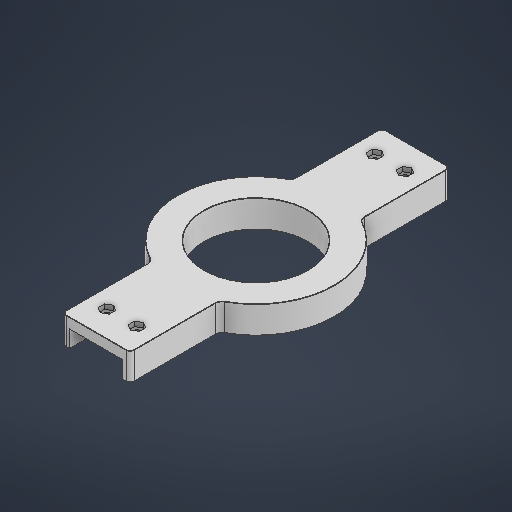
# Autodesk Inventor part: Head Thing
Saved by Autodesk Inventor 2025 (Build 290162000, 162)
## iProperties
Created: 2024-04-28
Part Number: Head Thing
Material: Generic
Document SubType Name: Modeling
Designer: Thienan Hoang
Density: 1 g/cm^3
Appearance: Default
Author: Thienan Hoang
Autodesk Inventor part; units mm, degrees
ref_plane "YZ Plane" through (0, 0, 0) normal (1, 0, 0) x (0, 1, 0)
ref_plane "XZ Plane" through (0, 0, 0) normal (0, 1, 0) x (-1, 0, 0)
ref_plane "XY Plane" through (0, 0, 0) normal (0, 0, 1) x (1, 0, 0)
sketch "Sketch1" plane through (0, 0, 0) normal (0, 1, 0) x (-1, 0, 0)
  circle A0 centre (0, 0) radius 38.125
  line L0 (25, 117.5) -> (-25, 117.5)
  line L1 (-25, -117.5) -> (25, -117.5)
  arc A1 (-25, 51.7808) -> (-25, -51.7808) centre (0, 0) ccw
  arc A2 (25, -51.7808) -> (25, 51.7808) centre (0, 0) ccw
  line L2 (-25, 117.5) -> (-25, 51.7808)
  line L3 (-25, -51.7808) -> (-25, -117.5)
  line L4 (25, -117.5) -> (25, -51.7808)
  line L5 (25, 51.7808) -> (25, 117.5)
  dimension "d0" = 76.25
  dimension "d76" = 50
  dimension "d77" = 57.5
  dimension "d78" = 57.5
  dimension "d79" = 65.7192
  dimension "d80" = 65.7192
  dimension "d81" = 50
  dimension "d82" = 235
  constraints: 12 end point, 5 parallel, 4 point on circle, 3 centre point, 2 coincident, 2 perpendicular, 1 horizontal
  measures "d0" diameter of A0
  measures "d76" distance between parallel lines of L5 L2
  measures "d77" radius of A1
  measures "d78" radius of A2
  measures "d79" distance of L5.start L0.start
  measures "d80" distance of L1.end L4.end
  measures "d81" distance of L1.start L1.end
  measures "d82" distance between parallel lines of L1 L0
extrude "Extrusion1" add sketch "Sketch1" along normal blind 20
fillet "Fillet1" radius 5 4 edges at (-25, 10, 51.7808) (25, 10, 51.7808) (25, 10, -51.7808) (-25, 10, -51.7808)
fillet "Fillet2" radius 3 4 edges at (25, 10, 117.5) (-25, 10, 117.5) (25, 10, -117.5) (-25, 10, -117.5)
chamfer "Chamfer1" distance 0.25 angle 45 34 edges at (25, 20, 84.6646) (25.6988, 20, 52.2798) (57.5, 20, 0) (25.6988, 20, -52.2798) (25, 20, -84.6646) (24.1213, 20, -116.6213) (0, 20, -117.5) (-24.1213, 20, -116.6213) (-25, 20, -84.6646) (-25.6988, 20, -52.2798) (-57.5, 20, 0) (-25.6988, 20, 52.2798) (-25, 20, 84.6646) (-24.1213, 20, 116.6213) (0, 20, 117.5) (24.1213, 20, 116.6213) (25, 0, 84.6646) (25.6988, 0, 52.2798) (57.5, 0, 0) (25.6988, 0, -52.2798) (25, 0, -84.6646) (24.1213, 0, -116.6213) (0, 0, -117.5) (-24.1213, 0, -116.6213) (-25, 0, -84.6646) (-25.6988, 0, -52.2798) (-57.5, 0, 0) (-25.6988, 0, 52.2798) (-25, 0, 84.6646) (-24.1213, 0, 116.6213) (0, 0, 117.5) (24.1213, 0, 116.6213) (38.125, 20, 0) (38.125, 0, 0)
sketch "Sketch3" plane through (0, 0, 0) normal (0, -1, 0) x (1, 0, 0)
  line L0 (-22, -117.25) -> (-22, 117.25)
  line L1 (22, 117.25) -> (22, -117.25)
  line L2 (22, -117.25) -> (-22, 117.25) construction
  line L3 (-22, -117.25) -> (22, 117.25) construction
  line L4 (16.625, 89) -> (-16.625, 89)
  line L5 (-19.625, 92) -> (-19.625, 117.25)
  line L6 (19.625, 117.25) -> (19.625, 92)
  line L7 (19.625, 89) -> (17.4099, 92.7868) construction
  line L8 (-19.625, 89) -> (-17.1837, 91.5811) construction
  line L9 (-19.625, -117.25) -> (-19.625, -91.9916)
  line L10 (-16.6334, -88.9916) -> (16.6165, -88.8986)
  line L11 (19.6248, -91.8986) -> (19.6248, -117.25)
  line L12 (-17.2012, -91.6745) -> (-19.625, -89) construction
  line L13 (17.2501, -91.935) -> (19.6248, -88.8902) construction
  line L14 (22, 117.25) -> (19.625, 117.25)
  line L15 (-22, 117.5) -> (22, 117.5) projected
  line L16 (-19.625, 117.25) -> (-22, 117.25)
  arc A0 (-16.6334, -88.9916) -> (-19.625, -91.9916) centre (-16.625, -91.9916) ccw
  arc A1 (19.6248, -91.8986) -> (16.6165, -88.8986) centre (16.6248, -91.8986) ccw
  arc A2 (-19.625, 92) -> (-16.625, 89) centre (-16.625, 92) ccw
  arc A3 (16.625, 89) -> (19.625, 92) centre (16.625, 92) ccw
  line L17 (19.6248, -117.25) -> (19.6248, -121.1164)
  line L18 (19.6248, -121.1164) -> (-19.625, -121.1164)
  line L19 (-19.625, -121.1164) -> (-19.625, -117.25)
  line L20 (19.625, 117.25) -> (19.625, 123.825)
  line L21 (19.625, 123.825) -> (-19.625, 123.825)
  line L22 (-19.625, 123.825) -> (-19.625, 117.25)
  line L23 (19.625, 117.25) -> (19.6248, 117.25)
  line L24 (22, -117.25) -> (19.6248, -117.25)
  line L25 (-19.625, -117.25) -> (-22, -117.25)
  point P0 (0, 0)
  point P1 (-19.625, 117.5)
  point P2 (19.625, 117.5)
  dimension "d35" = 39.25
  dimension "d37" = 28.25
  dimension "d38" = 28.25
  dimension "d39" = 39.25
  dimension "d40" = 3
  dimension "d41" = 3
  dimension "d42" = 3
  dimension "d50" = 2.375
  dimension "d51" = 2.375
  dimension "d52" = 44
  dimension "d53" = 39.2499
  dimension "d55" = 2.3752
  dimension "d56" = 2.375
  dimension "d83" = 234.5
  constraints: 50 end point, 14 point on line, 9 perpendicular, 8 point on circle, 8 tangent, 5 parallel, 4 centre point, 3 horizontal, 2 midpoint, 1 collinear, 1 equal radius, 1 vertical
  measures "d35" distance of L12.end L13.end
  measures "d37" distance of L9.start L12.end
  measures "d38" distance of L8.start L5.end
  measures "d39" distance of L7.start L8.start
  measures "d40" radius of A0
  measures "d41" radius of A1
  measures "d42" radius of A2
  measures "d50" distance between parallel lines of L6 L1
  measures "d51" distance between parallel lines of L0 L5
  measures "d52" distance between parallel lines of L0 L1
  measures "d53" distance between parallel lines of L19 L17
  measures "d55" distance between parallel lines of L11 L1
  measures "d56" distance between parallel lines of L0 L9
  measures "d83" distance of L0.start L0.end
extrude "Extrusion4" cut sketch "Sketch3" against normal blind 12.575 contours L9 A0 L10 A1 L11 L17 L18 L19 | L22 L15 L20 L6 A3 L4 A2 L5 | L22 L21 L20 L15
sketch "Sketch4" plane through (0, 12.575, 0) normal (0, -1, 0) x (1, 0, 0)
  circle A0 centre (11, 98.5) radius 2.2451
  circle A1 centre (-11, 98.5) radius 2.3292
  circle A2 centre (10.9998, -98.5) radius 1.5784
  circle A3 centre (-11.0002, -98.5) radius 2.3162
  line L0 (19.6248, -117.5) -> (-19.625, -117.5) projected
  line L1 (-19.625, -117.5) -> (-19.625, -91.9916) projected
  line L2 (19.6248, -91.8986) -> (19.6248, -117.5) projected
  line L3 (-19.625, 117.5) -> (19.625, 117.5) projected
  line L4 (19.625, 117.25) -> (19.625, 92) projected
  point P0 (0, 0)
  point P1 (-19.625, -117.25)
  point P2 (19.6248, -117.25)
  dimension "d45" = 19
  dimension "d48" = 19
  dimension "d57" = 19
  dimension "d58" = 19
  dimension "d59" = 22
  dimension "d60" = 22
  dimension "d61" = 8.625
  dimension "d62" = 8.625
  constraints: 4 centre point
  measures "d45" distance from line of L0 A3.centre
  measures "d48" distance from line of L0 A2.centre
  measures "d57" distance from line of L3 A0.centre
  measures "d58" distance from line of L3 A1.centre
  measures "d59" distance of A1.centre A0.centre
  measures "d60" distance of A3.centre A2.centre
  measures "d61" distance from line of L2 A2.centre
  measures "d62" distance from line of L4 A0.centre
hole "Hole2" at (11, 12.575, 98.5) at (-11, 12.575, 98.5) at (10.9998, 12.575, -98.5) at (-11.0002, 12.575, -98.5) direction (0, 1, 0) diameter 4.134 end through all thread size "M5x0.8" class "6H" standard "ANSI Metric M Profile"
sketch "Sketch5" plane through (0, 20, 0) normal (0, 1, 0) x (1, 0, 0)
  circle A0 centre (-11, -98.5) radius 2.067 projected
  line L0 (-11, -93.7369) -> (-6.875, -96.1184)
  line L1 (-6.875, -96.1184) -> (-6.875, -100.8816)
  line L2 (-6.875, -100.8816) -> (-11, -103.2631)
  line L3 (-11, -103.2631) -> (-15.125, -100.8816)
  line L4 (-15.125, -100.8816) -> (-15.125, -96.1184)
  line L5 (-15.125, -96.1184) -> (-11, -93.7369)
  circle A1 centre (11, -98.5) radius 2.067 projected
  line L6 (11, -93.7369) -> (15.125, -96.1184)
  line L7 (15.125, -96.1184) -> (15.125, -100.8816)
  line L8 (15.125, -100.8816) -> (11, -103.2631)
  line L9 (11, -103.2631) -> (6.875, -100.8816)
  line L10 (6.875, -100.8816) -> (6.875, -96.1184)
  line L11 (6.875, -96.1184) -> (11, -93.7369)
  circle A2 centre (-11.0002, 98.5) radius 2.067 projected
  line L12 (-11.0002, 93.7369) -> (-15.1252, 96.1184)
  line L13 (-15.1252, 96.1184) -> (-15.1252, 100.8816)
  line L14 (-15.1252, 100.8816) -> (-11.0002, 103.2631)
  line L15 (-11.0002, 103.2631) -> (-6.8752, 100.8816)
  line L16 (-6.8752, 100.8816) -> (-6.8752, 96.1184)
  line L17 (-6.8752, 96.1184) -> (-11.0002, 93.7369)
  circle A3 centre (10.9998, 98.5) radius 2.067 projected
  line L18 (10.9998, 103.2631) -> (15.1248, 100.8816)
  line L19 (15.1248, 100.8816) -> (15.1248, 96.1184)
  line L20 (15.1248, 96.1184) -> (10.9998, 93.7369)
  line L21 (10.9998, 93.7369) -> (6.8748, 96.1184)
  line L22 (6.8748, 96.1184) -> (6.8748, 100.8816)
  line L23 (6.8748, 100.8816) -> (10.9998, 103.2631)
  point P0 (0, 0)
  point P1 (-13.0625, -102.0724)
  point P2 (-8.9377, 94.9276)
  dimension "d70" = 8.25
  dimension "d71" = 8.25
  dimension "d72" = 8.25
  dimension "d73" = 8.25
  constraints: 48 end point, 4 coincident, 2 midpoint, 52 other
  measures "d70" distance from line of L0 point (-13.062, -102.072)
  measures "d71" distance from line of point (-8.938, 94.928) L14
  measures "d72" distance between parallel lines of L20 L23
  measures "d73" distance between parallel lines of L8 L11
extrude "Extrusion5" cut sketch "Sketch5" against normal blind 3.45
sketch "Sketch6" plane through (0, 0, 0) normal (0, -1, 0) x (1, 0, 0)
  circle A0 centre (0, 0) radius 41.25
  circle A1 centre (0, -41.25) radius 2.5
  circle A2 centre (41.25, 0) radius 2.5
  circle A3 centre (0, 41.25) radius 2.5
  circle A4 centre (-41.25, 0) radius 2.5
  dimension "d84" = 82.5
  dimension "d85" = 5
  dimension "d88" = 360
  constraints: 4 centre point, 1 coincident, 1 vertical alignment, 11 other
  measures "d85" diameter of A1
extrude "Extrusion6" cut sketch "Sketch6" against normal blind 3 contours A0 A2 | A0 A2 | A3 A0 | A0 A3 | A1 A0 | A0 A1 | A4 A0 | A0 A4
body "Solid1"
